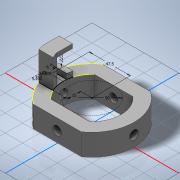
# Autodesk Inventor part: Part3
Saved by Autodesk Inventor 2022 (Build 260153000, 153)
## iProperties
Created: 2021-09-22
Part Number: Part3
Material: Generic
Document SubType Name: Modeling
Designer: WASHINGTON
Density: 1 g/cm^3
Appearance: Default
Author: WASHINGTON
Autodesk Inventor part; units mm, degrees
ref_plane "YZ Plane" through (0, 0, 0) normal (1, 0, 0) x (0, 1, 0)
ref_plane "XZ Plane" through (0, 0, 0) normal (0, 1, 0) x (-1, 0, 0)
ref_plane "XY Plane" through (0, 0, 0) normal (0, 0, 1) x (1, 0, 0)
sketch "Sketch1" plane through (0, 0, 0) normal (0, 1, 0) x (-1, 0, 0)
  line L0 (-22.2991, -25) -> (22.2991, -25)
  line L1 (22.2991, 25) -> (-22.2991, 25)
  arc A0 (-22.2991, 25) -> (-22.2991, -25) centre (0, 0) ccw
  arc A1 (22.2991, -25) -> (22.2991, 25) centre (0, 0) ccw
  line L2 (27.4272, 40) -> (-27.4272, 40)
  line L3 (27.4272, -40) -> (-27.4272, -40)
  arc A2 (27.4272, -40) -> (27.4272, 40) centre (0, 0) ccw
  arc A3 (-27.4272, 40) -> (-27.4272, -40) centre (0, 0) ccw
  dimension "d2" = 50
  dimension "d3" = 33.5
  dimension "d4" = 33.5
  dimension "d5" = 44.5982
  dimension "d7" = 15
  dimension "d8" = 15
  dimension "d9" = 48.5
  dimension "d10" = 48.5
  constraints: 8 end point, 8 point on circle, 4 centre point, 3 horizontal, 2 coincident, 1 parallel
  measures "d2" distance between parallel lines of L0 L1
  measures "d3" radius of A0
  measures "d4" radius of A1
  measures "d5" distance of L0.start L0.end
  measures "d7" distance between parallel lines of L1 L2
  measures "d8" distance between parallel lines of L3 L0
  measures "d9" radius of A2
  measures "d10" radius of A3
extrude "Extrusion1" add sketch "Sketch1" along normal mid plane 25
sketch "Sketch3" plane through (0, 0, 0) normal (0, 0, 1) x (1, 0, 0)
  circle A0 centre (0, 0) radius 5
  dimension "d13" = 10
  constraints: 1 centre point, 1 coincident
  measures "d13" diameter of A0
extrude "Extrusion2" cut sketch "Sketch3" along normal through all both and the other way through all
sketch "Sketch5" plane through (0, 0, 0) normal (1, 0, 0) x (0, 1, 0)
  circle A0 centre (0, 0) radius 5
  dimension "d17" = 10
  constraints: 1 centre point, 1 coincident
  measures "d17" diameter of A0
extrude "Extrusion3" cut sketch "Sketch5" along normal through all both and the other way through all
sketch "Sketch6" plane through (0, 12.5, 0) normal (0, 1, 0) x (1, 0, 0)
  circle A0 centre (0, 0) radius 25 construction
  arc A1 (-22.2991, 25) -> (-22.2991, -25) centre (0, 0) ccw projected
  line L0 (-33.5, 0) -> (-47.5, 0) construction
  line L1 (-46.1221, -15) -> (-29.9541, -15)
  line L2 (-31.9726, 10) -> (-47.4579, 10)
  arc A2 (-27.4272, 40) -> (-27.4272, -40) centre (0, 0) ccw projected
  arc A3 (-47.4579, 10) -> (-47.4986, 9.8046) centre (0, 0) ccw
  line L3 (-32.5308, -8) -> (-47.8357, -8)
  arc A4 (-33.5, 0) -> (-29.9541, -15) centre (0, 0) ccw
  arc A5 (-47.5, -9.798) -> (-46.1221, -15) centre (0, 0) ccw
  arc A6 (-47.4579, 10) -> (-47.5, -9.798) centre (0, 0) ccw
  arc A7 (-31.9726, 10) -> (-33.5, 0) centre (0, 0) ccw
  line L4 (-48.2416, 5) -> (-33.1248, 5) projected
  arc A8 (-22.2991, 25) -> (-22.2991, -25) centre (0, 0) ccw projected
  line L5 (-33.2603, 4) -> (-48.3348, 4)
  dimension "d25" = 50
  dimension "d26" = 25
  dimension "d27" = 7
  dimension "d28" = 15
  dimension "d29" = 15
  dimension "d30" = 24.8046
  dimension "d31" = 5.202
  dimension "d32" = 47.5
  dimension "d37" = 6
  constraints: 21 point on circle, 10 end point, 6 centre point, 6 coincident, 3 parallel, 2 concentric, 2 horizontal, 2 other
  measures "d25" diameter of A0
  measures "d26" distance between parallel lines of L2 L1
  measures "d27" distance between parallel lines of L3 L1
  measures "d28" distance between parallel lines of L0 L1
  measures "d29" distance from line of point (0, 0) L1
  measures "d30" distance from line of A3.end L1
  measures "d31" distance from line of A5.start L1
  measures "d32" distance of A1.centre L0.end
  measures "d37" distance between parallel lines of L2 L5
extrude "Extrusion4" add sketch "Sketch6" along normal blind 6 contours A1 L4 A2 L2 | A1 L5 A2 L4 | A1 L3 A2 L5
extrude "Extrusion5" add sketch "Sketch6" along normal blind 33 contours A1 L1 A2 L3
extrude "Extrusion6" cut sketch "Sketch6" along normal through all contours A1 L3 A2 L5
sketch "Sketch7" plane through (-32.5308, 45.5, 8) normal (0, 0, -1) x (-1, 0, 0)
  line L0 (0, 0) -> (15.3049, 0) projected
  line L1 (-2.5766, -33) -> (-2.5766, 0) projected
  line L2 (15.3049, 0) -> (0, 0)
  line L3 (0, -5) -> (15.3049, -5)
  line L4 (15.3049, -5) -> (15.3049, 0)
  line L5 (0, 0) -> (0, -5)
  line L6 (0, -33) -> (0, 0) projected
  point P0 (-32.5308, -45.5)
  dimension "d40" = 5
  dimension "d41" = 15.3049
  constraints: 8 end point, 2 point on line, 1 horizontal, 1 parallel
  measures "d40" distance of L3.end L0.end
  measures "d41" distance of L3.start L3.end
extrude "Extrusion7" add sketch "Sketch7" along normal up to surface (18 mm away)
body "Solid1"
